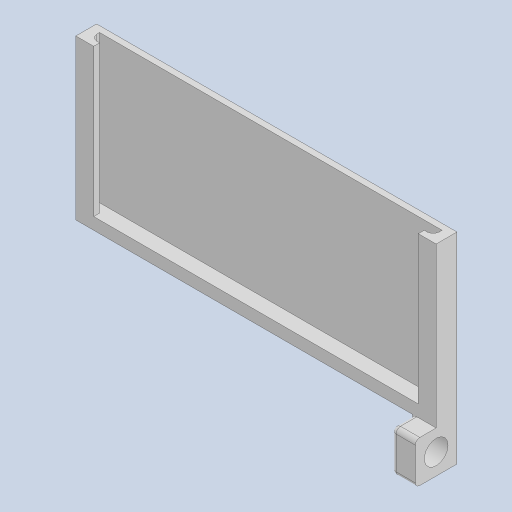
# Autodesk Inventor part: RFID_holder_PCB_01
Saved by Autodesk Inventor 2024.4 (Build 284460000, 460)
## iProperties
Created: 2026-03-24
Part Number: RFID_holder_PCB_01
Material: Generic
Document SubType Name: Modeling
Designer: Admin
Density: 1 g/cm^3
Appearance: Default
Author: Admin
Autodesk Inventor part; units mm, degrees
ref_plane "YZ Plane" through (0, 0, 0) normal (1, 0, 0) x (0, 1, 0)
ref_plane "XZ Plane" through (0, 0, 0) normal (0, 1, 0) x (-1, 0, 0)
ref_plane "XY Plane" through (0, 0, 0) normal (0, 0, 1) x (1, 0, 0)
derived "PCB.ipt"
sketch "Sketch1: PCB" plane through (0, 0, 0) normal (0, 0, 1) x (1, 0, 0)
  line L0 (-22.0554, 53.3935) -> (34.5446, 53.3935)
  line L1 (34.5446, 53.3935) -> (34.5446, 28.5935)
  line L2 (34.5446, 28.5935) -> (-22.0554, 28.5935)
  line L3 (-22.0554, 28.5935) -> (-22.0554, 53.3935)
  line L4 (2.3446, 55.1935) -> (9.9446, 55.1935)
  line L5 (9.9446, 55.1935) -> (9.9446, 45.9935)
  line L6 (9.9446, 45.9935) -> (2.3446, 45.9935)
  line L7 (2.3446, 45.9935) -> (2.3446, 55.1935)
  point P0 (0, 0)
sketch "Sketch3: PCB base & outside walls" plane through (0, 0, 0) normal (0, 0, 1) x (1, 0, 0)
  line L0 (-22.0554, 28.5935) -> (-22.0554, 53.3935) construction
  line L1 (-22.0554, 53.3935) -> (34.5446, 53.3935) construction
  line L2 (34.5446, 28.5935) -> (-22.0554, 28.5935) construction
  line L3 (34.5446, 53.3935) -> (34.5446, 28.5935) construction
  line L4 (-24.0554, 53.3935) -> (36.5446, 53.3935)
  line L5 (36.5446, 53.3935) -> (36.5446, 26.5935)
  line L6 (36.5446, 26.5935) -> (-24.0554, 26.5935)
  line L7 (-24.0554, 26.5935) -> (-24.0554, 53.3935)
  line L8 (35.0446, 53.3935) -> (35.0446, 28.5935)
  line L9 (35.0446, 28.5935) -> (-22.5554, 28.5935)
  line L10 (-22.5554, 28.5935) -> (-22.5554, 53.3935)
  point P0 (0, 0)
  dimension "d28" = 2
  dimension "d31" = 0.5
  dimension "d32" = 0.5
  dimension "d45" = 1.5
  dimension "d46" = 1.5
  dimension "d53" = 57.6
  constraints: 14 end point, 2 collinear, 2 point on line
  measures "d28" distance between parallel lines of L6 L2
  measures "d31" distance between parallel lines of L0 L10
  measures "d32" distance between parallel lines of L8 L3
  measures "d45" distance between parallel lines of L10 L7
  measures "d46" distance between parallel lines of L5 L8
  measures "d53" distance between parallel lines of L8 L10
sketch "Sketch4: PCB slider" plane through (0, 0, 0) normal (0, 0, 1) x (1, 0, 0)
  line L0 (-21.0554, 53.3935) -> (-21.0554, 28.5935)
  line L1 (33.5446, 53.3935) -> (33.5446, 28.5935)
  line L2 (-24.0554, 53.3935) -> (36.5446, 53.3935) projected
  line L3 (35.0446, 28.5935) -> (-22.5554, 28.5935) projected
  line L4 (-22.0554, 28.5935) -> (-22.0554, 53.3935) construction
  line L5 (34.5446, 53.3935) -> (34.5446, 28.5935) construction
  line L6 (35.0446, 53.3935) -> (35.0446, 28.5935) projected
  line L7 (-22.5554, 28.5935) -> (-22.5554, 53.3935) projected
  point P0 (0, 0)
  dimension "d33" = 1
  dimension "d34" = 1
  constraints: 4 end point, 4 point on line
  measures "d33" distance between parallel lines of L0 L4
  measures "d34" distance between parallel lines of L5 L1
sketch "Sketch8: extra piece" plane through (0, 0, 0) normal (0, 0, 1) x (1, 0, 0)
  line L0 (36.5446, 19.5935) -> (32.5446, 19.5935)
  line L1 (32.5446, 19.5935) -> (32.5446, 26.5935)
  line L2 (36.5446, 26.5935) -> (36.5446, 19.5935)
  line L3 (36.5446, 26.5935) -> (-24.0554, 26.5935) construction
  line L4 (36.5446, 53.3935) -> (36.5446, 26.5935) construction
  line L5 (36.5446, 26.5935) -> (32.5446, 26.5935)
  point P0 (0, 0)
  dimension "d61" = 7
  dimension "d62" = 4
  constraints: 8 end point, 2 collinear, 2 perpendicular
  measures "d61" distance of L0.end L1.end
  measures "d62" distance of L0.start L0.end
extrude "Ex4: PCB base" add sketch "Sketch3: PCB base & outside walls" along normal blind 1
extrude "Ex5: PCB outside walls" add sketch "Sketch3: PCB base & outside walls" along normal blind 3.5 contours L4 L10 L9 L8 L5 L6 L7
extrude "Ex6: PCB slider" add sketch "Sketch4: PCB slider" against normal blind 1 from surface at 3.5 contours L0 L3 L7 L2 | L2 L6 L3 L1
fillet "Fillet1" radius 1 2 edges at (-22.5554, 40.9935, 2.5) (35.0446, 40.9935, 2.5)
extrude "Ex9: extra piece" add sketch "Sketch8: extra piece" along normal blind 7
sketch "Sketch9: heat set" plane through (36.5446, 53.3935, 3.5) normal (1, 0, 0) x (0, 0, -1)
  circle A0 centre (0, -30.3) radius 2
  line L0 (3.5, -33.8) -> (-3.5, -33.8) projected
  line L1 (-3.5, -33.8) -> (-3.5, -26.8) projected
  point P0 (3.5, -53.3935)
  point P1 (0, -33.8)
  point P2 (-3.5, -30.3)
  dimension "d60" = 4
  constraints: 2 midpoint, 1 centre point, 1 horizontal alignment, 1 vertical alignment
  measures "d60" diameter of A0
extrude "Ex10: heat set" cut sketch "Sketch9: heat set" against normal through all
fillet "Fillet2" radius 0.75 5 edges at (34.5446, 19.5935, 7) (32.5446, 19.5935, 3.5) (32.5446, 23.0935, 7) (32.5446, 26.5935, 5.25) (34.5446, 26.5935, 7)
equation "\"d32\" = d31"
equation "\"d46\" = d45"
body "Solid1"
